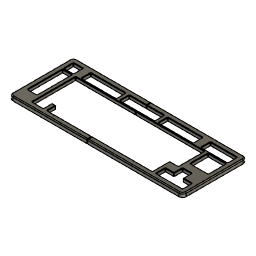
KBO-5000-Case-Redesign-UpperPart (Autodesk Fusion 360 design; units mm, degrees)
Autodesk Fusion 360 part; units mm, degrees
other "Base Mesh Feature1"
other "Modify7"
other "Modify9"
other "Base Mesh Feature2"
other "Modify8"
other "Modify10"
sketch "Right-TopDown" plane through (0, 0, 0) normal (0, 0, 1) x (1, 0, 0)
  line L0 (212.025, 0) -> (212.025, 143.063)
  line L1 (0, 0) -> (0, 11.05)
  line L2 (212.025, 143.063) -> (0, 143.063)
  line L3 (0, 0) -> (212.025, 0)
  line L4 (0, 143.063) -> (0, 132.013)
  line L5 (0, 132.013) -> (38.575, 132.013)
  line L6 (38.575, 132.013) -> (38.575, 111.538)
  line L7 (38.575, 111.538) -> (0, 111.538)
  line L8 (0, 111.538) -> (0, 107.725)
  line L9 (0, 107.725) -> (152.875, 107.725)
  line L10 (152.875, 107.725) -> (152.875, 49.625)
  line L11 (152.875, 49.625) -> (133.825, 49.625)
  line L12 (133.825, 49.625) -> (133.825, 11.05)
  line L13 (133.825, 11.05) -> (0, 11.05)
  line L14 (200.975, 111.538) -> (142.4, 111.538)
  line L15 (200.975, 111.538) -> (200.975, 132.013)
  line L16 (200.975, 132.013) -> (142.4, 132.013)
  line L17 (142.4, 132.013) -> (142.4, 111.538)
  line L18 (124.3, 111.538) -> (47.15, 111.538)
  line L19 (47.15, 111.538) -> (47.15, 132.013)
  line L20 (47.15, 132.013) -> (124.3, 132.013)
  line L21 (124.3, 132.013) -> (124.3, 111.538)
  line L22 (161.45, 31.525) -> (142.4, 31.525)
  line L23 (142.4, 31.525) -> (142.4, 11.05)
  line L24 (142.4, 11.05) -> (200.975, 11.05)
  line L25 (200.975, 11.05) -> (200.975, 31.525)
  line L26 (200.975, 31.525) -> (181.45, 31.525)
  line L27 (181.45, 31.525) -> (181.45, 50.575)
  line L28 (181.45, 50.575) -> (161.45, 50.575)
  line L29 (161.45, 50.575) -> (161.45, 31.525)
  line L30 (161.45, 107.725) -> (200.975, 107.725)
  line L31 (200.975, 107.725) -> (200.975, 68.2)
  line L32 (200.975, 68.2) -> (161.45, 68.2)
  line L33 (161.45, 68.2) -> (161.45, 107.725)
  dimension "d1" = 212.025
  dimension "d3" = 11.05
  dimension "d5" = 212.025
  dimension "d6" = 143.063
  dimension "d14" = 11.05
  dimension "d15" = 38.575
  dimension "d16" = 20.475
  dimension "d17" = 3.813
  dimension "d18" = 152.875
  dimension "d19" = 58.1
  dimension "d20" = 19.05
  dimension "d21" = 38.575
  dimension "d25" = 20.475
  dimension "d26" = 58.575
  dimension "d27" = 11.05
  dimension "d28" = 8.575
  dimension "d29" = 18.1
  dimension "d34" = 19.05
  dimension "d35" = 20.475
  dimension "d36" = 58.575
  dimension "d37" = 20.475
  dimension "d38" = 19.525
  dimension "d39" = 19.05
  dimension "d93" = 11.05
  dimension "d96" = 8.575
  dimension "d97" = 39.525
  dimension "d98" = 39.525
  constraint vertical L0
  constraint coincident L1.start L3.start
  constraint horizontal L3
  constraint horizontal L2
  constraint perpendicular L2 L4
  constraint perpendicular L4 L5
  constraint perpendicular L5 L6
  constraint perpendicular L6 L7
  constraint perpendicular L7 L8
  constraint perpendicular L8 L9
  constraint perpendicular L9 L10
  constraint perpendicular L10 L11
  constraint perpendicular L11 L12
  constraint perpendicular L1 L13
  constraint vertical L15
  constraint horizontal L16
  constraint vertical L17
  constraint horizontal L18
  constraint vertical L19
  constraint horizontal L20
  constraint vertical L21
  constraint perpendicular L22 L23
  constraint perpendicular L23 L24
  constraint perpendicular L24 L25
  constraint perpendicular L25 L26
  constraint perpendicular L26 L27
  constraint perpendicular L22 L29
  constraint horizontal L30
  constraint vertical L31
  constraint horizontal L32
  constraint vertical L33
  measures "d1" distance of L1.start L0.start
  measures "d3" distance of L1.start L1.end
  measures "d5" distance of L1.start L0.start
  measures "d6" distance of L1.start L2.end
  measures "d14" distance of L2.end L4.end
  measures "d15" distance of L4.end L5.end
  measures "d16" distance of L5.end L6.end
  measures "d17" distance of L7.end L8.end
  measures "d18" distance of L8.end L9.end
  measures "d19" distance of L9.end L10.end
  measures "d20" distance of L10.end L11.end
  measures "d21" distance of L11.end L12.end
  measures "d25" distance of L15.end L14.start
  measures "d26" distance of L14.start L14.end
  measures "d27" distance of L2 L16
  measures "d28" distance of L5.end L19.end
  measures "d29" distance of L14.end L18.start
  measures "d34" distance of L22.start L22.end
  measures "d35" distance of L22.end L23.end
  measures "d36" distance of L23.end L24.end
  measures "d37" distance of L24.end L25.end
  measures "d38" distance of L25.end L26.end
  measures "d39" distance of L26.end L27.end
  measures "d93" distance of L0 L25
  measures "d96" distance of L9.end L30.start
  measures "d97" distance of L30.start L30.end
  measures "d98" distance of L30.start L32.end
sketch "Right-BottomEdge" plane through (0, 0, 0) normal (0, 0, 1) x (1, 0, 0)
  line L0 (0, 0) -> (212.025, 0)
  line L1 (212.025, 0) -> (212.025, 143.063)
  line L2 (212.025, 143.063) -> (0, 143.063)
  line L3 (0, 143.063) -> (0, 139.313)
  line L4 (0, 0) -> (0, 3.75)
  line L5 (0, 139.313) -> (208.275, 139.313)
  line L6 (0, 3.75) -> (208.275, 3.75)
  line L7 (208.275, 139.313) -> (208.275, 3.75)
  circle A0 centre (203.4392, 134.4767) radius 1.65
  circle A1 centre (143.35, 135.0625) radius 1.65
  circle A2 centre (123.35, 135.0625) radius 1.65
  circle A3 centre (52.8625, 135.0625) radius 1.65
  circle A4 centre (32.8625, 135.0625) radius 1.65
  circle A5 centre (4, 135.0625) radius 1.65
  circle A6 centre (203.4392, 8.5857) radius 1.65
  circle A7 centre (103.0125, 8) radius 1.65
  circle A8 centre (4, 8) radius 1.65
  dimension "d59" = 212.025
  dimension "d60" = 143.063
  dimension "d61" = 212.025
  dimension "d62" = 3.75
  dimension "d63" = 3.75
  dimension "d64" = 208.275
  dimension "d65" = 208.275
  dimension "d121" = 3.3
  dimension "d122" = 3.3
  dimension "d123" = 3.3
  dimension "d124" = 3.3
  dimension "d125" = 3.3
  dimension "d126" = 3.3
  dimension "d127" = 3.3
  dimension "d128" = 3.3
  dimension "d129" = 3.3
  constraint coincident L0.start L4.start
  constraint horizontal L0
  constraint perpendicular L0 L1
  constraint perpendicular L1 L2
  constraint perpendicular L2 L3
  constraint perpendicular L0 L4
  constraint perpendicular L3 L5
  constraint perpendicular L4 L6
  measures "d59" distance of L0.start L0.end
  measures "d60" distance of L0.end L1.end
  measures "d61" distance of L1.end L2.end
  measures "d62" distance of L2.end L3.end
  measures "d63" distance of L0.start L4.end
  measures "d64" distance of L3.end L5.end
  measures "d65" distance of L4.end L6.end
  measures "d121" diameter of A0
  measures "d122" diameter of A1
  measures "d123" diameter of A2
  measures "d124" diameter of A3
  measures "d125" diameter of A4
  measures "d126" diameter of A5
  measures "d127" diameter of A8
  measures "d128" diameter of A7
  measures "d129" diameter of A6
sketch "Left-TopDown" plane through (0, 0, 0) normal (0, 0, 1) x (1, 0, 0)
  line L0 (0, 0) -> (-173.925, 0)
  line L1 (-173.925, 0) -> (-173.925, 143.063)
  line L2 (-173.925, 143.063) -> (0, 143.063)
  line L3 (0, 143.063) -> (0, 132.013)
  line L4 (0, 0) -> (0, 11.05)
  line L5 (0, 132.013) -> (-38.575, 132.013)
  line L6 (-38.575, 132.013) -> (-38.575, 111.538)
  line L7 (-38.575, 111.538) -> (0, 111.538)
  line L8 (0, 111.538) -> (0, 107.725)
  line L9 (0, 107.725) -> (-133.825, 107.725)
  line L10 (-133.825, 107.725) -> (-133.825, 11.05)
  line L11 (-133.825, 11.05) -> (-109.063, 11.05)
  line L12 (-109.063, 11.05) -> (-109.063, 30.575)
  line L13 (-109.063, 30.575) -> (-100.488, 30.575)
  line L14 (-100.488, 30.575) -> (-100.488, 11.05)
  line L15 (-100.488, 11.05) -> (0, 11.05)
  line L16 (-47.15, 111.538) -> (-124.3, 111.538)
  line L17 (-124.3, 111.538) -> (-124.3, 132.013)
  line L18 (-124.3, 132.013) -> (-47.15, 132.013)
  line L19 (-47.15, 132.013) -> (-47.15, 111.538)
  line L20 (-142.4, 107.725) -> (-162.875, 107.725)
  line L21 (-162.875, 107.725) -> (-162.875, 30.1)
  line L22 (-162.875, 30.1) -> (-142.4, 30.1)
  line L23 (-142.4, 30.1) -> (-142.4, 107.725)
  line L24 (-162.875, 111.538) -> (-142.4, 111.538)
  line L25 (-142.4, 111.538) -> (-142.4, 132.013)
  line L26 (-142.4, 132.013) -> (-162.875, 132.013)
  line L27 (-162.875, 132.013) -> (-162.875, 111.538)
  dimension "d68" = 173.925
  dimension "d69" = 143.063
  dimension "d70" = 173.925
  dimension "d71" = 11.05
  dimension "d72" = 11.05
  dimension "d73" = 38.575
  dimension "d74" = 20.475
  dimension "d75" = 38.575
  dimension "d76" = 3.813
  dimension "d77" = 133.825
  dimension "d78" = 96.675
  dimension "d79" = 24.762
  dimension "d80" = 19.525
  dimension "d81" = 8.575
  dimension "d82" = 19.525
  dimension "d83" = 8.575
  dimension "d84" = 77.15
  dimension "d85" = 20.475
  dimension "d86" = 8.575
  dimension "d87" = 20.475
  dimension "d88" = 77.625
  dimension "d90" = 3.813
  dimension "d91" = 20.475
  dimension "d92" = 20.475
  constraint coincident L0.start L4.start
  constraint horizontal L0
  constraint perpendicular L0 L1
  constraint perpendicular L1 L2
  constraint perpendicular L2 L3
  constraint vertical L4
  constraint perpendicular L3 L5
  constraint perpendicular L5 L6
  constraint perpendicular L6 L7
  constraint perpendicular L7 L8
  constraint horizontal L9
  constraint perpendicular L9 L10
  constraint perpendicular L10 L11
  constraint perpendicular L11 L12
  constraint perpendicular L12 L13
  constraint perpendicular L13 L14
  constraint horizontal L16
  constraint vertical L17
  constraint horizontal L18
  constraint vertical L19
  constraint horizontal L20
  constraint vertical L21
  constraint horizontal L22
  constraint vertical L23
  constraint horizontal L24
  constraint vertical L25
  constraint horizontal L26
  constraint vertical L27
  measures "d68" distance of L0.start L0.end
  measures "d69" distance of L0.end L1.end
  measures "d70" distance of L1.end L2.end
  measures "d71" distance of L2.end L3.end
  measures "d72" distance of L0.start L4.end
  measures "d73" distance of L3.end L5.end
  measures "d74" distance of L5.end L6.end
  measures "d75" distance of L6.end L7.end
  measures "d76" distance of L7.end L8.end
  measures "d77" distance of L8.end L9.end
  measures "d78" distance of L9.end L10.end
  measures "d79" distance of L10.end L11.end
  measures "d80" distance of L11.end L12.end
  measures "d81" distance of L12.end L13.end
  measures "d82" distance of L13.end L14.end
  measures "d83" distance of L6.end L16.start
  measures "d84" distance of L16.start L16.end
  measures "d85" distance of L16.start L18.end
  measures "d86" distance of L9.end L20.start
  measures "d87" distance of L20.start L20.end
  measures "d88" distance of L20.start L22.end
  measures "d90" distance of L20.end L24.start
  measures "d91" distance of L24.start L24.end
  measures "d92" distance of L24.start L26.end
sketch "Left-BottomEdge" plane through (0, 0, 0) normal (0, 0, 1) x (1, 0, 0)
  line L0 (0, 0) -> (-173.925, 0)
  line L1 (-173.925, 0) -> (-173.925, 143.063)
  line L2 (-173.925, 143.063) -> (0, 143.063)
  line L3 (0, 143.063) -> (0, 139.313)
  line L4 (0, 0) -> (0, 3.75)
  line L5 (0, 139.313) -> (-170.175, 139.313)
  line L6 (0, 3.75) -> (-170.175, 3.75)
  line L7 (-170.175, 139.313) -> (-170.175, 3.75)
  circle A0 centre (-4, 135.0625) radius 1.65
  circle A1 centre (-32.8625, 135.0625) radius 1.65
  circle A2 centre (-52.8625, 135.0625) radius 1.65
  circle A3 centre (-123.35, 135.0625) radius 1.65
  circle A4 centre (-143.35, 135.0625) radius 1.65
  circle A5 centre (-165.3392, 134.4767) radius 1.65
  circle A6 centre (-165.3392, 8.5858) radius 1.65
  circle A7 centre (-83.9625, 8) radius 1.65
  circle A8 centre (-4, 8) radius 1.65
  dimension "d101" = 173.925
  dimension "d102" = 143.063
  dimension "d103" = 173.925
  dimension "d104" = 3.75
  dimension "d105" = 3.75
  dimension "d106" = 170.175
  dimension "d107" = 170.175
  dimension "d112" = 3.3
  dimension "d113" = 3.3
  dimension "d114" = 3.3
  dimension "d115" = 3.3
  dimension "d116" = 3.3
  dimension "d117" = 3.3
  dimension "d118" = 3.3
  dimension "d119" = 3.3
  dimension "d120" = 3.3
  constraint coincident L0.start L4.start
  constraint horizontal L0
  constraint perpendicular L0 L1
  constraint perpendicular L1 L2
  constraint perpendicular L2 L3
  constraint perpendicular L0 L4
  constraint horizontal L5
  constraint perpendicular L4 L6
  measures "d101" distance of L0.start L0.end
  measures "d102" distance of L0.end L1.end
  measures "d103" distance of L1.end L2.end
  measures "d104" distance of L2.end L3.end
  measures "d105" distance of L0.start L4.end
  measures "d106" distance of L3.end L5.end
  measures "d107" distance of L4.end L6.end
  measures "d112" diameter of A0
  measures "d113" diameter of A1
  measures "d114" diameter of A2
  measures "d115" diameter of A3
  measures "d116" diameter of A4
  measures "d117" diameter of A5
  measures "d118" diameter of A8
  measures "d119" diameter of A7
  measures "d120" diameter of A6
extrude "Extrude-Right-Main" add sketch "Right-TopDown" along normal blind 7 makes body 1
move_body "Move1" bodies 1 to x (1, 0, 0) y (0, 1, 0) z (0, 0, 1) at (0, 0, 1.7)
extrude "Extrude-Right-Foot" add sketch "Right-BottomEdge" along normal blind 1.7 contours L0 L1 L2 L3 L4 L5 L6 L7 bodies 1
extrude "Extrude-Right-ScrewSpace" cut sketch "Right-BottomEdge" along normal blind 7 contours A0 | A1 | A2 | A3 | A4 | A5 | A6 | A7 | A8 bodies 1
fillet "Fillet-Right-Inner" radius 1 63 edges at (19.2875, 132.013, 8.7) (85.725, 132.013, 8.7) (47.15, 121.7755, 8.7) (38.575, 121.7755, 8.7) (19.2875, 111.538, 8.7) (85.725, 111.538, 8.7) (124.3, 121.7755, 8.7) (171.6875, 132.013, 8.7) (142.4, 121.7755, 8.7) (200.975, 121.7755, 8.7) (171.6875, 111.538, 8.7) (161.45, 87.9625, 8.7) (181.2125, 107.725, 8.7) (200.975, 87.9625, 8.7) (181.2125, 68.2, 8.7) (171.45, 50.575, 8.7) (161.45, 41.05, 8.7) (151.925, 31.525, 8.7) (142.4, 21.2875, 8.7) (171.6875, 11.05, 8.7) (200.975, 21.2875, 8.7) (191.2125, 31.525, 8.7) (181.45, 41.05, 8.7) (76.4375, 107.725, 8.7) (152.875, 78.675, 8.7) (143.35, 49.625, 8.7) (133.825, 30.3375, 8.7) (66.9125, 11.05, 8.7) (0, 137.538, 8.7) (0, 132.013, 5.2) (0, 109.6315, 8.7) (0, 111.538, 5.2) (0, 107.725, 5.2) (0, 5.525, 8.7) (0, 11.05, 5.2) (0, 0, 4.35) (0, 143.063, 4.35) (38.575, 132.013, 5.2) (38.575, 111.538, 5.2) (47.15, 132.013, 5.2) (47.15, 111.538, 5.2) (124.3, 132.013, 5.2) (124.3, 111.538, 5.2) (200.975, 132.013, 5.2) (200.975, 111.538, 5.2) (142.4, 132.013, 5.2) (142.4, 111.538, 5.2) (200.975, 107.725, 5.2) (161.45, 107.725, 5.2) (161.45, 68.2, 5.2) (200.975, 68.2, 5.2) (161.45, 50.575, 5.2) (181.45, 50.575, 5.2) (181.45, 31.525, 5.2) (200.975, 31.525, 5.2) (200.975, 11.05, 5.2) (142.4, 11.05, 5.2) (142.4, 31.525, 5.2) (161.45, 31.525, 5.2) (152.875, 107.725, 5.2) (152.875, 49.625, 5.2) (133.825, 49.625, 5.2) (133.825, 11.05, 5.2) on bodies 1
fillet "Fillet-Right-OuterEdge" radius 2 5 edges at (106.5125, 143.063, 8.7) (0.2929, 142.7701, 8.4071) (212.025, 71.5315, 8.7) (0.2929, 0.2929, 8.4071) (106.5125, 0, 8.7) on bodies 1
fillet "Fillet-Right-OuterCorner" radius 8 4 edges at (212.025, 0, 3.35) (211.4392, 0.5858, 8.1142) (212.025, 143.063, 3.35) (211.4392, 142.4772, 8.1142) on bodies 1
fillet "Fillet-Right-FootCorner" radius 4.25 2 edges at (208.275, 139.313, 0.85) (208.275, 3.75, 0.85) on bodies 1
extrude "Extrude-Left-Main" add sketch "Left-TopDown" along normal blind 7 separate body makes body 2
move_body "Move2" bodies 2 to x (1, 0, 0) y (0, 1, 0) z (0, 0, 1) at (0, 0, 1.7)
extrude "Extrude-Left-Foot" add sketch "Left-BottomEdge" along normal blind 1.7 contours L0 L1 L2 L3 L4 L5 L6 L7 bodies 2
extrude "Extrude-Left-ScrewSpace" cut sketch "Left-BottomEdge" along normal blind 7 contours A0 | A1 | A2 | A3 | A4 | A5 | A6 | A7 | A8 bodies 2
fillet "Fillet-Left-Inner" radius 1 51 edges at (-152.6375, 132.013, 8.7) (-142.4, 121.7755, 8.7) (-162.875, 121.7755, 8.7) (-152.6375, 111.538, 8.7) (-162.875, 68.9125, 8.7) (-152.6375, 107.725, 8.7) (-142.4, 68.9125, 8.7) (-152.6375, 30.1, 8.7) (-124.3, 121.7755, 8.7) (-85.725, 132.013, 8.7) (-47.15, 121.7755, 8.7) (-85.725, 111.538, 8.7) (-19.2875, 132.013, 8.7) (-38.575, 121.7755, 8.7) (-19.2875, 111.538, 8.7) (0, 137.538, 8.7) (0, 143.063, 4.35) (0, 132.013, 5.2) (-38.575, 132.013, 5.2) (-38.575, 111.538, 5.2) (0, 109.6315, 8.7) (0, 111.538, 5.2) (0, 107.725, 5.2) (-66.9125, 107.725, 8.7) (-133.825, 59.3875, 8.7) (-133.825, 107.725, 5.2) (-121.444, 11.05, 8.7) (-109.063, 20.8125, 8.7) (-104.7755, 30.575, 8.7) (-100.488, 20.8125, 8.7) (-50.244, 11.05, 8.7) (0, 11.05, 5.2) (0, 5.525, 8.7) (0, 0, 4.35) (-100.488, 30.575, 5.2) (-109.063, 30.575, 5.2) (-109.063, 11.05, 5.2) (-133.825, 11.05, 5.2) (-124.3, 132.013, 5.2) (-47.15, 132.013, 5.2) (-47.15, 111.538, 5.2) (-124.3, 111.538, 5.2) (-142.4, 132.013, 5.2) (-162.875, 132.013, 5.2) (-162.875, 111.538, 5.2) (-142.4, 111.538, 5.2) (-142.4, 30.1, 5.2) (-162.875, 30.1, 5.2) (-162.875, 107.725, 5.2) (-142.4, 107.725, 5.2) (-100.488, 11.05, 5.2) on bodies 2
fillet "Fillet-Left-OuterEdge" radius 2 5 edges at (-87.4625, 0, 8.7) (-0.2929, 0.2929, 8.4071) (-173.925, 71.5315, 8.7) (-0.2929, 142.7701, 8.4071) (-87.4625, 143.063, 8.7) on bodies 2
fillet "Fillet-Left-OuterCorner" radius 8 4 edges at (-173.925, 0, 3.35) (-173.3392, 0.5858, 8.1142) (-173.925, 143.063, 3.35) (-173.3392, 142.4772, 8.1142) on bodies 2
fillet "Fillet-Left-FootCorner" radius 4.25 2 edges at (-170.175, 3.75, 0.85) (-170.175, 139.313, 0.85) on bodies 2
named bodies: "RightPart", "LeftPart"
